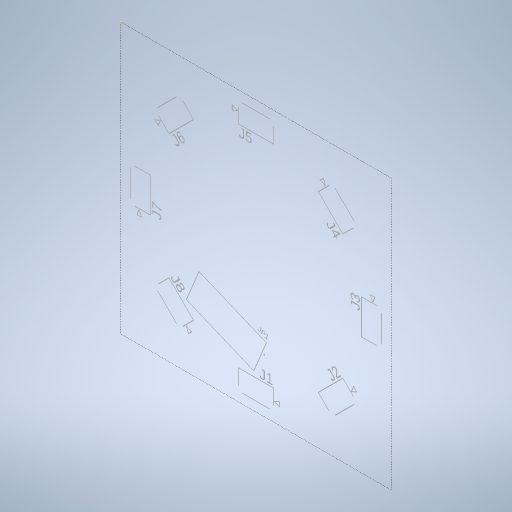
# Autodesk Inventor part: Clippard 8-MC 3D PCB Top
Saved by Autodesk Inventor 2024.2 (Build 282272000, 272)
## iProperties
Created: 2024-03-21
Part Number: Clippard 8-MC 3D PCB Top
Material: Generic
Document SubType Name: Modeling
Designer: shann
Density: 1 g/cm^3
Appearance: Clear - Light
Author: shann
Autodesk Inventor part; units mm, degrees
ref_plane "YZ Plane" through (0, 0, 0) normal (1, 0, 0) x (0, 1, 0)
ref_plane "XZ Plane" through (0, 0, 0) normal (0, 1, 0) x (-1, 0, 0)
ref_plane "XY Plane" through (0, 0, 0) normal (0, 0, 1) x (1, 0, 0)
sketch "Sketch1" plane through (0, 0, 0) normal (0, 0, 1) x (1, 0, 0)
  line L0 (0, 0) -> (75.184, 0)
  line L1 (75.184, 0) -> (75.184, -75.184)
  line L2 (75.184, -75.184) -> (0, -75.184)
  line L3 (0, -75.184) -> (0, 0)
  dimension "d5" = 75.184
  constraints: 1 coincident, 1 horizontal, 2 other
  measures "d5" distance of L2.end L0.start
extrude "Extrusion1" add sketch "Sketch1" along normal blind 0.254
sketch "Sketch2" plane through (0, 0, 0) normal (0, 0, 1) x (1, 0, 0)
  line L0 (22.0209, 0) -> (53.1631, 0)
  line L1 (53.1631, 0) -> (75.184, -22.0209)
  line L2 (75.184, -22.0209) -> (75.184, -53.1631)
  line L3 (75.184, -53.1631) -> (53.1631, -75.184)
  line L4 (53.1631, -75.184) -> (22.0209, -75.184)
  line L5 (22.0209, -75.184) -> (0, -53.1631)
  line L6 (0, -53.1631) -> (0, -22.0209)
  line L7 (0, -22.0209) -> (22.0209, 0)
  line L8 (0, 0) -> (75.184, 0) projected
  line L9 (0, -75.184) -> (0, 0) projected
  line L10 (75.184, -75.184) -> (0, -75.184) projected
  line L11 (75.184, 0) -> (75.184, -75.184) projected
  line L12 (0, 0) -> (0, -75.184) projected
  line L13 (0, -75.184) -> (75.184, -75.184) projected
  point P0 (53.1631, 0)
  point P1 (0, -53.1631)
  dimension "d13" = 135
  dimension "d14" = 135
  dimension "d15" = 135
  dimension "d16" = 135
  constraints: 16 end point, 5 equal length, 4 point on line, 2 horizontal, 2 vertical
  measures "d13" angle of L7 L0
  measures "d14" angle of L1 L0
  measures "d15" angle of L5 L6
  measures "d16" angle of L4 L3
extrude "Extrusion2" cut sketch "Sketch2" along normal mid plane 25.4 contours L7 L9 L8 | L8 L11 L1 | L5 L10 L9 | L11 L10 L3
sketch "Sketch3" plane through (0, 0, 0) normal (0, 0, 1) x (1, 0, 0)
  line L0 (0, 0) -> (75.184, 0) construction
  line L1 (75.184, 0) -> (75.184, -75.184) construction
  line L2 (75.184, -75.184) -> (0, -75.184) construction
  line L3 (0, -75.184) -> (0, 0) construction
  line L4 (53.1631, -75.184) -> (22.0209, -75.184) construction
  line L5 (0, -53.1631) -> (0, -22.0209) construction
  line L6 (22.0209, 0) -> (53.1631, 0) construction
  point P0 (0, 0)
  constraints: 3 collinear, 1 horizontal, 2 other
equation "\"d14\" = d13"
equation "\"d15\" = d13"
equation "\"d16\" = d14"
body "Solid1"
